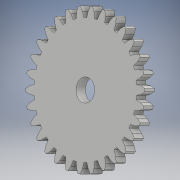
# Autodesk Inventor part: Колесо
Saved by Autodesk Inventor 2018.1 (Build 221171000, 171)
## iProperties
Part Number: Колесо
Material: Типовые
Document SubType Name: Modeling
Designer: Пугачева Екатерина
Density: 1 g/cm^3
Appearance: По умолчанию
Mass: 13.5094 g
Surface Area: 74.3038 cm^2
Volume: 13.5094 cm^3
Author: Пугачева Екатерина
Autodesk Inventor part; units mm, degrees
ref_plane "YZ Plane" through (0, 0, 0) normal (1, 0, 0) x (0, 1, 0)
ref_plane "XZ Plane" through (0, 0, 0) normal (0, 1, 0) x (-1, 0, 0)
ref_plane "XY Plane" through (0, 0, 0) normal (0, 0, 1) x (1, 0, 0)
sketch "Эскиз1" plane through (0, 0, 0) normal (0, 0, 1) x (1, 0, 0)
  line L0 (0, 0) -> (0, 5)
  line L1 (5, 5) -> (32, 5)
  line L2 (32, 5) -> (32, 0)
  line L3 (32, 0) -> (5, 0)
  line L4 (5, 0) -> (5, 5)
  dimension "d0" = 5
  dimension "d1" = 10
  dimension "d2" = 5
  dimension "d3" = 64
  constraints: 10 end point, 2 parallel, 1 horizontal, 1 perpendicular, 1 point on line, 1 vertical
  measures "d0" distance of L0.start L0.end
  measures "d1" diameter of L4 L0
  measures "d2" distance of L1.end L2.end
  measures "d3" diameter of L2 L0
revolve "Вращение1" add sketch "Эскиз1" angle 360 about axis through (0, 0, 0) along (0, 1, 0)
sketch "Эскиз2" plane through (0, 5, 0) normal (0, 1, 0) x (1, 0, 0)
  circle A0 centre (0, 0) radius 30 construction
  circle A1 centre (0, 0) radius 27.5 construction
  line L0 (-0.785, 27.4888) -> (0.785, 27.4888)
  line L1 (-0.785, 27.4888) -> (-1.57, 29.9589)
  line L2 (-1.57, 29.9589) -> (-2.7475, 31.8818)
  circle A2 centre (0, 0) radius 32 projected
  line L3 (0.785, 27.4888) -> (1.57, 29.9589)
  line L4 (2.7475, 31.8818) -> (1.57, 29.9589)
  dimension "d5" = 60
  dimension "d6" = 55
  dimension "d7" = 1.57
  dimension "d8" = 3.14
  dimension "d9" = 5.495
  constraints: 10 end point, 6 point on circle, 2 centre point, 2 coincident, 2 equal length, 1 horizontal
  measures "d5" diameter of A0
  measures "d6" diameter of A1
  measures "d7" distance of L0.start L0.end
  measures "d8" distance of L3.end L1.end
  measures "d9" distance of L4.start L2.end
extrude "Выдавливание1" cut sketch "Эскиз2" against normal up to next contours L1 L2 A2 L4 L3 L0 picked at (-0.2617, 29.1355)
pattern_circular "Круговой массив1" count 30 over 360 about axis through (0, -10, 0) along (0, 1, 0) of "Выдавливание1"
